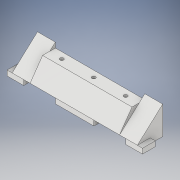
# Autodesk Inventor part: sameSpacer
Saved by Autodesk Inventor 2019 (Build 230136000, 136)
## iProperties
Created: 2020-12-06
Part Number: sameSpacer
Material: Пластик АБС
Document SubType Name: Modeling
Designer: Professional
Density: 1.06 g/cm^3
Appearance: Гладкий — белый
Author: Professional
Autodesk Inventor part; units mm, degrees
ref_plane "YZ Plane" through (0, 0, 0) normal (1, 0, 0) x (0, 1, 0)
ref_plane "XZ Plane" through (0, 0, 0) normal (0, 1, 0) x (-1, 0, 0)
ref_plane "XY Plane" through (0, 0, 0) normal (0, 0, 1) x (1, 0, 0)
sketch "Эскиз1" plane through (0, 0, 0) normal (0, 1, 0) x (-1, 0, 0)
  line L0 (0, 0) -> (10, 0)
  line L1 (10, 0) -> (10, -4)
  line L2 (10, -4) -> (30, -4)
  line L3 (30, -4) -> (30, 0)
  line L4 (30, 0) -> (49, 0)
  line L5 (49, 0) -> (49, 9.8)
  line L6 (49, 9.8) -> (53, 9.8)
  line L7 (53, 9.8) -> (53, 19.8)
  line L8 (53, 19.8) -> (40, 19.8)
  line L9 (40, 19.8) -> (40, 15.8)
  line L10 (40, 15.8) -> (15, 15.8)
  line L11 (15, 15.8) -> (15, 19.8)
  line L12 (15, 19.8) -> (0, 19.8)
  line L13 (0, 19.8) -> (0, 0)
  line L14 (0, 0) -> (-10, 0)
  line L15 (-10, 0) -> (-10, -4)
  line L16 (-10, -4) -> (-30, -4)
  line L17 (-30, -4) -> (-30, 0)
  line L18 (-30, 0) -> (-49, 0)
  line L19 (-49, 0) -> (-49, 9.8)
  line L20 (-49, 9.8) -> (-53, 9.8)
  line L21 (-53, 9.8) -> (-53, 19.8)
  line L22 (-53, 19.8) -> (-40, 19.8)
  line L23 (-40, 19.8) -> (-40, 15.8)
  line L24 (-40, 15.8) -> (-15, 15.8)
  line L25 (-15, 15.8) -> (-15, 19.8)
  line L26 (-15, 19.8) -> (0, 19.8)
  dimension "d0" = 20
  dimension "d1" = 4
  dimension "d2" = 20
  dimension "d3" = 19
  dimension "d4" = 19.8
  dimension "d5" = 30
  dimension "d6" = 25
  dimension "d7" = 10
  constraints: 54 end point, 12 symmetric about line, 11 perpendicular, 8 point on line, 2 equal length, 1 horizontal
  measures "d0" distance of L1.end L2.end
  measures "d1" distance of L2.end L3.end
  measures "d2" diameter of L1 L13
  measures "d3" distance of L3.end L4.end
  measures "d4" distance between parallel lines of L8 L4
  measures "d5" diameter of L11 L13
  measures "d6" distance between parallel lines of L9 L11
  measures "d7" distance between parallel lines of L8 L6
extrude "Выдавливание1" add sketch "Эскиз1" along normal blind 4
sketch "Эскиз3" plane through (49, 0, 9.8) normal (1, 0, 0) x (0, 0, -1)
  line L0 (-10, 4) -> (0, 4) projected
  line L1 (-10, 4) -> (9.8, 22)
  line L2 (9.8, 4) -> (13.8, 4) projected
  line L3 (9.8, 22) -> (9.8, 4)
  line L4 (0, 0) -> (9.8, 0) projected
  line L5 (-10, 4) -> (9.8, 4)
  dimension "d10" = 22
  constraints: 6 end point, 1 collinear, 1 perpendicular
  measures "d10" distance from line of L1.end L4
extrude "Выдавливание2" add sketch "Эскиз3" against normal up to surface (98 mm away)
sketch "Эскиз6" plane through (10, 0, 0) normal (0, 0, -1) x (-1, 0, 0)
  line L0 (-39, 22) -> (59, 22) projected
  line L1 (-25, 22) -> (45, 22)
  line L2 (45, 22) -> (45, 18)
  line L3 (45, 18) -> (-25, 18)
  line L4 (-25, 18) -> (-25, 22)
  line L5 (0, 0) -> (20, 0) projected
  point P0 (10, 0)
  point P1 (10, 18)
  point P2 (10, 0)
  dimension "d13" = 70
  dimension "d14" = 4
  constraints: 8 end point, 2 midpoint, 2 parallel, 1 horizontal, 1 perpendicular, 1 point on line, 1 vertical alignment
  measures "d13" distance between parallel lines of L2 L4
  measures "d14" distance between parallel lines of L0 L3
extrude "Выдавливание3" cut sketch "Эскиз6" against normal through all
sketch "Эскиз8" plane through (35, 18, 0) normal (-1, 0, 0) x (0, 0, 1)
  line L0 (0, 4) -> (4.4, 0) projected
  line L1 (0, 0) -> (0, 4) projected
  line L2 (0, 0) -> (4.4, 0) projected
  line L3 (4.4, 0) -> (10, 0)
  line L4 (19.8, -18) -> (19.8, -14) projected
  line L5 (10, 0) -> (19.8, -14)
  line L6 (19.8, -14) -> (4.4, 0)
  line L7 (19.8, -14) -> (0, 4) projected
  line L8 (0, -18) -> (0, 4) projected
  dimension "d17" = 10
  constraints: 6 end point, 1 collinear, 1 horizontal
  measures "d17" distance from line of L8 L3.end
extrude "Выдавливание4" add sketch "Эскиз8" along normal up to surface (70 mm away) contours L3 L5 L6
sketch "Эскиз10" plane through (-35, 18, 0) normal (0, 1, 0) x (1, 0, 0)
  line L0 (35, 0) -> (35, -10)
  line L1 (70, -10) -> (0, -10) projected
  point P0 (60, -5)
  point P1 (35, -5)
  point P2 (10, -5)
  dimension "d27" = 5
  dimension "d28" = 50
  constraints: 2 end point, 2 horizontal alignment, 2 midpoint, 1 symmetric about line
  measures "d27" distance from line of L1 point (60, -5)
  measures "d28" distance of point (10, -5) point (60, -5)
hole "Отверстие1" at (25, 18, 5) at (0, 18, 5) at (-25, 18, 5) direction (0, -1, 0) diameter 2.8 depth 8
